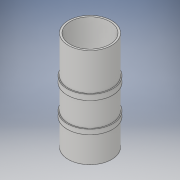
# Autodesk Inventor part: Flaschenhalter
Saved by Autodesk Inventor 2019 (Build 230136000, 136)
## iProperties
Created: 2019-02-21
Part Number: Flaschenhalter
Material: Generisch
Document SubType Name: Modeling
Designer: nico-
Density: 1 g/cm^3
Appearance: Vorgabe
Author: nico-
Autodesk Inventor part; units mm, degrees
ref_plane "YZ Plane" through (0, 0, 0) normal (1, 0, 0) x (0, 1, 0)
ref_plane "XZ Plane" through (0, 0, 0) normal (0, 1, 0) x (-1, 0, 0)
ref_plane "XY Plane" through (0, 0, 0) normal (0, 0, 1) x (1, 0, 0)
sketch "Skizze1" plane through (0, 0, 0) normal (0, 1, 0) x (-1, 0, 0)
  circle A0 centre (0, 0) radius 32.1
  circle A1 centre (0, 0) radius 35
  dimension "d0" = 64.2
  dimension "d1" = 70
  constraints: 2 centre point, 2 coincident
  measures "d0" diameter of A0
  measures "d1" diameter of A1
extrude "Extrusion1" add sketch "Skizze1" along normal blind 160
sketch "Skizze3" plane through (0, 0, 0) normal (1, 0, 0) x (0, 1, 0)
  line L0 (100, 34.6803) -> (91, 34.6803)
  line L1 (0, 32.1) -> (160, 32.1) projected
  line L2 (100, 34.6803) -> (109, 34.6803) construction
  line L3 (91, 34.6803) -> (91, 36.6803)
  line L4 (91, 36.6803) -> (100, 36.6803)
  line L5 (100, 36.6803) -> (100, 34.6803)
  line L6 (0, 35) -> (160, 35) projected
  line L7 (51, 35) -> (42, 35)
  line L8 (42, 35) -> (43.0847, 36.6803)
  line L9 (43.0847, 36.6803) -> (51, 36.6803)
  line L10 (51, 36.6803) -> (51, 35)
  line L11 (0, 0) -> (162.7697, 0)
  line L12 (160, -35) -> (160, 35) projected
  dimension "d4" = 9
  dimension "d5" = 180
  dimension "d6" = 2
  dimension "d7" = 9
  dimension "d8" = 2
  dimension "d10" = 60
  dimension "d11" = 40
  constraints: 20 end point, 4 perpendicular, 4 point on line, 2 horizontal, 1 collinear, 1 parallel
  measures "d4" distance of L0.start L0.end
  measures "d5" angle of L0 L2
  measures "d6" distance of L0.end L3.end
  measures "d7" distance of L7.start L7.end
  measures "d8" distance of L7.end L8.end
  measures "d10" distance from line of L12 L0.start
  measures "d11" distance from line of L9.end L3
revolve "Umdrehung1" add sketch "Skizze3" angle 360 about axis through (0, 0, 0) along (0, 1, 0)
